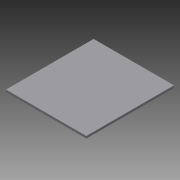
# Autodesk Inventor part: Front
Saved by Autodesk Inventor 2015 (Build 190159000, 159)
## iProperties
Created: 2018-04-13
Part Number: Front
Material: Generic
Document SubType Name: Modeling
Designer: Toby
Density: 1 g/cm^3
Appearance: Default
Author: Toby
Autodesk Inventor part; units mm, degrees
ref_plane "YZ Plane" through (0, 0, 0) normal (1, 0, 0) x (0, 1, 0)
ref_plane "XZ Plane" through (0, 0, 0) normal (0, 1, 0) x (-1, 0, 0)
ref_plane "XY Plane" through (0, 0, 0) normal (0, 0, 1) x (1, 0, 0)
sketch "Sketch1" plane through (0, 0, 0) normal (0, 0, 1) x (1, 0, 0)
  line L0 (-43.5457, 39.1136) -> (-3.5457, 39.1136)
  line L1 (-3.5457, 39.1136) -> (-3.5457, -4.8864)
  line L2 (-3.5457, -4.8864) -> (-43.5457, -4.8864)
  line L3 (-43.5457, -4.8864) -> (-43.5457, 39.1136)
  point P0 (0, 0)
  dimension "d0" = 40
  dimension "d1" = 44
  constraints: 8 end point, 2 parallel, 1 horizontal, 1 perpendicular
  measures "d0" distance of L0.start L0.end
  measures "d1" distance of L2.end L0.start
extrude "Extrusion1" add sketch "Sketch1" along normal blind 1.2
sketch "Sketch2" plane through (0, 0, 1.2) normal (0, 0, 1) x (1, 0, 0)
  line L0 (-45.5457, 41.1136) -> (-1.5457, 41.1136)
  line L1 (-1.5457, 41.1136) -> (-1.5457, -6.8864)
  line L2 (-1.5457, -6.8864) -> (-45.5457, -6.8864)
  line L3 (-45.5457, -6.8864) -> (-45.5457, 41.1136)
  line L4 (-3.5457, 39.1136) -> (-43.5457, 39.1136) projected
  line L5 (-43.5457, -4.8864) -> (-3.5457, -4.8864) projected
  line L6 (-3.5457, -4.8864) -> (-3.5457, 39.1136) projected
  line L7 (-43.5457, 39.1136) -> (-43.5457, -4.8864) projected
  point P0 (0, 0)
  dimension "d4" = 2
  dimension "d5" = 2
  dimension "d6" = 2
  dimension "d7" = 2
  constraints: 8 end point, 2 parallel, 1 horizontal, 1 perpendicular
  measures "d4" distance between parallel lines of L4 L0
  measures "d5" distance between parallel lines of L2 L5
  measures "d6" distance between parallel lines of L1 L6
  measures "d7" distance between parallel lines of L7 L3
extrude "Extrusion2" add sketch "Sketch2" along normal blind 1.2 contours L0 L1 L2 L3 | L6 L5 L7 L4
body "Solid1"
